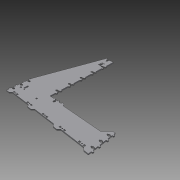
# Autodesk Inventor part: frame_left
Saved by Autodesk Inventor 2014 (Build 180170000, 170)
## iProperties
Created: 2013-12-03
Part Number: frame_left
Material: Generic
Document SubType Name: Modeling
Designer: buben
Density: 1 g/cm^3
Appearance: Default
Author: buben
Autodesk Inventor part; units mm, degrees
ref_plane "YZ Plane" through (0, 0, 0) normal (1, 0, 0) x (0, 1, 0)
ref_plane "XZ Plane" through (0, 0, 0) normal (0, 1, 0) x (-1, 0, 0)
ref_plane "XY Plane" through (0, 0, 0) normal (0, 0, 1) x (1, 0, 0)
sketch "Sketch1" plane through (0, 0, 0) normal (0, 0, 1) x (1, 0, 0)
  line L0 (0, 0) -> (489, 0)
  line L1 (489, 0) -> (489, 120)
  line L2 (0, 0) -> (0, 120)
  line L3 (0, 120) -> (111.5, 494)
  line L4 (111.5, 494) -> (161.5, 494)
  line L5 (161.5, 494) -> (161.5, 94)
  line L6 (489, 120) -> (479, 120)
  line L7 (479, 120) -> (449, 90)
  line L8 (449, 90) -> (251.5, 90)
  line L9 (251.5, 90) -> (241.5, 100)
  line L10 (241.5, 100) -> (231.5, 100)
  line L11 (231.5, 100) -> (231.5, 94)
  line L12 (231.5, 94) -> (161.5, 94)
  point P0 (244.5, 0)
  dimension "d0" = 489
  dimension "d1" = 83
  dimension "d2" = 120
  dimension "d3" = 45
  dimension "d5" = 6
  dimension "d6" = 70
  dimension "d7" = 10
  dimension "d8" = 10
  dimension "d9" = 50
  dimension "d10" = 494
  dimension "d13" = 10
  dimension "d15" = 20
  constraints: 26 end point, 7 perpendicular, 3 parallel, 1 horizontal, 1 horizontal alignment, 1 midpoint
  measures "d0" distance of L0.start L0.end
  measures "d1" distance from line of L5 point (244.5, 0)
  measures "d2" distance of L0.start L2.end
  measures "d3" angle of L6 L7
  measures "d5" distance of L10.end L11.end
  measures "d6" distance of L11.end L5.end
  measures "d7" distance of L1.end L6.end
  measures "d8" distance of L9.end L10.end
  measures "d9" distance of L3.end L4.end
  measures "d10" distance between parallel lines of L0 L4
  measures "d13" distance between parallel lines of L8 L10
  measures "d15" vertical distance of L2.end L10.end
extrude "Extrusion1" add sketch "Sketch1" along normal blind 6
sketch "Sketch2" plane through (0, 0, 6) normal (0, 0, 1) x (1, 0, 0)
  line L0 (0, 0) -> (489, 0) projected
  line L1 (489, 0) -> (489, 120) projected
  line L2 (251.5, 90) -> (241.5, 100) projected
  line L3 (489, 20.75) -> (489, 16.25)
  line L4 (472.7, 16.25) -> (472.7, 20.75)
  line L5 (476.7, 23.25) -> (484, 23.25)
  line L6 (484, 13.75) -> (476.7, 13.75)
  line L7 (472.7, 20.75) -> (476.7, 20.75)
  line L8 (484, 20.75) -> (489, 20.75)
  line L9 (489, 16.25) -> (484, 16.25)
  line L10 (476.7, 16.25) -> (472.7, 16.25)
  line L11 (476.7, 13.75) -> (476.7, 16.25)
  line L12 (476.7, 20.75) -> (476.7, 23.25)
  line L13 (484, 23.25) -> (484, 20.75)
  line L14 (484, 16.25) -> (484, 13.75)
  line L15 (489, 98.75) -> (489, 94.25)
  line L16 (472.7, 94.25) -> (472.7, 98.75)
  line L17 (476.7, 101.25) -> (484, 101.25)
  line L18 (484, 91.75) -> (476.7, 91.75)
  line L19 (472.7, 98.75) -> (476.7, 98.75)
  line L20 (484, 98.75) -> (489, 98.75)
  line L21 (489, 94.25) -> (484, 94.25)
  line L22 (476.7, 94.25) -> (472.7, 94.25)
  line L23 (476.7, 91.75) -> (476.7, 94.25)
  line L24 (476.7, 98.75) -> (476.7, 101.25)
  line L25 (484, 101.25) -> (484, 98.75)
  line L26 (484, 94.25) -> (484, 91.75)
  line L27 (489, 59.75) -> (489, 55.25)
  line L28 (472.7, 55.25) -> (472.7, 59.75)
  line L29 (476.7, 62.25) -> (484, 62.25)
  line L30 (484, 52.75) -> (476.7, 52.75)
  line L31 (472.7, 59.75) -> (476.7, 59.75)
  line L32 (484, 59.75) -> (489, 59.75)
  line L33 (489, 55.25) -> (484, 55.25)
  line L34 (476.7, 55.25) -> (472.7, 55.25)
  line L35 (476.7, 52.75) -> (476.7, 55.25)
  line L36 (476.7, 59.75) -> (476.7, 62.25)
  line L37 (484, 62.25) -> (484, 59.75)
  line L38 (484, 55.25) -> (484, 52.75)
  line L39 (244.5, 0) -> (244.5, 97) construction
  line L40 (0, 20.75) -> (0, 16.25)
  line L41 (16.3, 16.25) -> (16.3, 20.75)
  line L42 (12.3, 23.25) -> (5, 23.25)
  line L43 (5, 13.75) -> (12.3, 13.75)
  line L44 (16.3, 20.75) -> (12.3, 20.75)
  line L45 (5, 20.75) -> (0, 20.75)
  line L46 (0, 16.25) -> (5, 16.25)
  line L47 (12.3, 16.25) -> (16.3, 16.25)
  line L48 (12.3, 13.75) -> (12.3, 16.25)
  line L49 (12.3, 20.75) -> (12.3, 23.25)
  line L50 (5, 23.25) -> (5, 20.75)
  line L51 (5, 16.25) -> (5, 13.75)
  line L52 (16.3, 98.75) -> (12.3, 98.75)
  line L53 (16.3, 94.25) -> (16.3, 98.75)
  line L54 (12.3, 94.25) -> (16.3, 94.25)
  line L55 (12.3, 98.75) -> (12.3, 101.25)
  line L56 (12.3, 91.75) -> (12.3, 94.25)
  line L57 (12.3, 101.25) -> (5, 101.25)
  line L58 (5, 94.25) -> (5, 91.75)
  line L59 (5, 91.75) -> (12.3, 91.75)
  line L60 (5, 98.75) -> (0, 98.75)
  line L61 (0, 98.75) -> (0, 94.25)
  line L62 (0, 94.25) -> (5, 94.25)
  line L63 (5, 101.25) -> (5, 98.75)
  line L64 (12.3, 59.75) -> (12.3, 62.25)
  line L65 (16.3, 59.75) -> (12.3, 59.75)
  line L66 (16.3, 55.25) -> (16.3, 59.75)
  line L67 (12.3, 55.25) -> (16.3, 55.25)
  line L68 (12.3, 52.75) -> (12.3, 55.25)
  line L69 (12.3, 62.25) -> (5, 62.25)
  line L70 (5, 52.75) -> (12.3, 52.75)
  line L71 (5, 55.25) -> (5, 52.75)
  line L72 (5, 62.25) -> (5, 59.75)
  line L73 (0, 55.25) -> (5, 55.25)
  line L74 (5, 59.75) -> (0, 59.75)
  line L75 (0, 59.75) -> (0, 55.25)
  point P0 (472.7, 18.5)
  point P1 (480.35, 23.25)
  point P2 (472.7, 96.5)
  point P3 (480.35, 101.25)
  point P4 (472.7, 57.5)
  point P5 (480.35, 62.25)
  point P6 (16.3, 18.5)
  point P7 (8.65, 23.25)
  point P8 (16.3, 96.5)
  point P9 (8.65, 101.25)
  point P10 (16.3, 57.5)
  point P11 (8.65, 62.25)
  dimension "d16" = 4.5
  dimension "d17" = 2.5
  dimension "d18" = 2.5
  dimension "d19" = 4
  dimension "d20" = 7.3
  dimension "d21" = 5
  dimension "d23" = 4.5
  dimension "d24" = 2.5
  dimension "d25" = 2.5
  dimension "d26" = 4
  dimension "d27" = 7.3
  dimension "d28" = 5
  dimension "d30" = 4.5
  dimension "d31" = 2.5
  dimension "d32" = 2.5
  dimension "d33" = 4
  dimension "d34" = 7.3
  dimension "d35" = 5
  dimension "d40" = 18.5
  dimension "d41" = 39
  dimension "d42" = 39
  constraints: 146 end point, 42 symmetric about line, 30 parallel, 15 collinear, 13 perpendicular, 9 horizontal, 7 midpoint, 1 point on line
  measures "d16" distance of L4.start L4.end
  measures "d17" distance of L7.end L5.start
  measures "d18" distance of L6.end L10.start
  measures "d19" distance of L10.start L4.start
  measures "d20" distance of L6.start L6.end
  measures "d21" distance of L3.end L9.end
  measures "d23" distance of L16.start L19.start
  measures "d24" distance of L19.end L24.end
  measures "d25" distance of L23.start L22.start
  measures "d26" distance of L22.start L16.start
  measures "d27" distance of L26.end L23.start
  measures "d28" distance of L15.end L26.start
  measures "d30" distance of L28.start L31.start
  measures "d31" distance of L36.start L36.end
  measures "d32" distance of L35.start L34.start
  measures "d33" distance of L34.start L28.start
  measures "d34" distance of L30.start L35.start
  measures "d35" distance of L33.start L38.start
  measures "d40" distance from line of L0 point (472.7, 18.5)
  measures "d41" distance of point (472.7, 57.5) point (472.7, 18.5)
  measures "d42" distance of point (472.7, 57.5) point (472.7, 96.5)
extrude "Extrusion2" cut sketch "Sketch2" against normal through all
sketch "Sketch4" plane through (0, 0, 6) normal (0, 0, 1) x (1, 0, 0)
  line L0 (0, 16.25) -> (0, 0) projected
  line L1 (489, 0) -> (489, 16.25) projected
  line L2 (472.7, 16.25) -> (472.7, 20.75) projected
  line L3 (489, 20.75) -> (489, 55.25) projected
  line L4 (472.7, 55.25) -> (472.7, 59.75) projected
  line L5 (489, 59.75) -> (489, 94.25) projected
  line L6 (472.7, 94.25) -> (472.7, 98.75) projected
  line L7 (489, 98.75) -> (489, 120) projected
  line L8 (0, 120) -> (0, 98.75) projected
  line L9 (0, 94.25) -> (0, 59.75) projected
  line L10 (0, 55.25) -> (0, 20.75) projected
  line L11 (0, 112) -> (-4, 112)
  line L12 (-6, 110) -> (-6, 106)
  line L13 (-4, 104) -> (0, 104)
  line L14 (0, 104) -> (0, 112)
  line L15 (0, 81) -> (-4, 81)
  line L16 (-6, 79) -> (-6, 75)
  line L17 (-4, 73) -> (0, 73)
  line L18 (0, 73) -> (0, 81)
  line L19 (0, 42) -> (-4, 42)
  line L20 (-6, 40) -> (-6, 36)
  line L21 (-4, 34) -> (0, 34)
  line L22 (0, 34) -> (0, 42)
  line L23 (0, 11) -> (-4, 11)
  line L24 (-6, 9) -> (-6, 5)
  line L25 (-4, 3) -> (0, 3)
  line L26 (0, 3) -> (0, 11)
  line L27 (489, 112) -> (493, 112)
  line L28 (495, 110) -> (495, 106)
  line L29 (493, 104) -> (489, 104)
  line L30 (489, 104) -> (489, 112)
  line L31 (489, 81) -> (493, 81)
  line L32 (495, 79) -> (495, 75)
  line L33 (493, 73) -> (489, 73)
  line L34 (489, 73) -> (489, 81)
  line L35 (489, 42) -> (493, 42)
  line L36 (495, 40) -> (495, 36)
  line L37 (493, 34) -> (489, 34)
  line L38 (489, 34) -> (489, 42)
  line L39 (489, 11) -> (493, 11)
  line L40 (495, 9) -> (495, 5)
  line L41 (493, 3) -> (489, 3)
  line L42 (489, 3) -> (489, 11)
  arc A0 (-6, 5) -> (-4, 3) centre (-4, 5) ccw
  arc A1 (-4, 11) -> (-6, 9) centre (-4, 9) ccw
  arc A2 (-6, 36) -> (-4, 34) centre (-4, 36) ccw
  arc A3 (-4, 42) -> (-6, 40) centre (-4, 40) ccw
  arc A4 (-6, 75) -> (-4, 73) centre (-4, 75) ccw
  arc A5 (-4, 81) -> (-6, 79) centre (-4, 79) ccw
  arc A6 (-6, 106) -> (-4, 104) centre (-4, 106) ccw
  arc A7 (-4, 112) -> (-6, 110) centre (-4, 110) ccw
  arc A8 (495, 110) -> (493, 112) centre (493, 110) ccw
  arc A9 (493, 104) -> (495, 106) centre (493, 106) ccw
  arc A10 (495, 79) -> (493, 81) centre (493, 79) ccw
  arc A11 (493, 73) -> (495, 75) centre (493, 75) ccw
  arc A12 (495, 40) -> (493, 42) centre (493, 40) ccw
  arc A13 (493, 34) -> (495, 36) centre (493, 36) ccw
  arc A14 (495, 9) -> (493, 11) centre (493, 9) ccw
  arc A15 (493, 3) -> (495, 5) centre (493, 5) ccw
  line L43 (489, 20.75) -> (489, 55.25) projected
  point P0 (472.7, 96.5)
  point P1 (472.7, 57.5)
  point P2 (472.7, 18.5)
  point P3 (495, 77)
  point P4 (489, 77)
  point P5 (495, 38)
  point P6 (489, 38)
  dimension "d81" = 2
  dimension "d82" = 8
  dimension "d83" = 8
  dimension "d84" = 8
  dimension "d85" = 8
  dimension "d86" = 7.5
  dimension "d87" = 7.5
  dimension "d88" = 6
  dimension "d89" = 6
  constraints: 64 end point, 32 point on circle, 32 tangent, 16 centre point, 16 parallel, 15 equal radius, 14 collinear, 8 horizontal, 8 perpendicular, 8 point on line, 7 midpoint, 2 horizontal alignment
  measures "d81" radius of A0
  measures "d82" distance between parallel lines of L29 L27
  measures "d83" distance between parallel lines of L33 L31
  measures "d84" distance between parallel lines of L37 L35
  measures "d85" distance between parallel lines of L41 L39
  measures "d86" distance from line of point (472.7, 96.5) L29
  measures "d87" distance from line of point (472.7, 18.5) L39
  measures "d88" distance between parallel lines of L7 L28
  measures "d89" distance between parallel lines of L8 L12
extrude "Extrusion4" add sketch "Sketch4" against normal blind 6
sketch "Sketch5" plane through (0, 0, 6) normal (0, 0, 1) x (1, 0, 0)
  line L0 (231.5, 100) -> (231.5, 94) projected
  line L1 (231.5, 94) -> (161.5, 94) projected
  line L2 (199.75, 94) -> (204.25, 94)
  line L3 (204.25, 77.7) -> (199.75, 77.7)
  line L4 (206.75, 89) -> (206.75, 81.7)
  line L5 (197.25, 81.7) -> (197.25, 89)
  line L6 (204.25, 94) -> (204.25, 89)
  line L7 (204.25, 81.7) -> (204.25, 77.7)
  line L8 (199.75, 77.7) -> (199.75, 81.7)
  line L9 (199.75, 89) -> (199.75, 94)
  line L10 (197.25, 89) -> (199.75, 89)
  line L11 (204.25, 89) -> (206.75, 89)
  line L12 (206.75, 81.7) -> (204.25, 81.7)
  line L13 (199.75, 81.7) -> (197.25, 81.7)
  point P0 (202, 77.7)
  dimension "d92" = 4.5
  dimension "d93" = 2.5
  dimension "d94" = 2.5
  dimension "d95" = 5
  dimension "d96" = 7.3
  dimension "d97" = 4
  dimension "d98" = 29.5
  constraints: 24 end point, 10 parallel, 5 collinear, 4 perpendicular, 3 horizontal, 1 midpoint
  measures "d92" distance of L3.start L3.end
  measures "d93" distance of L8.end L5.start
  measures "d94" distance of L4.end L7.start
  measures "d95" distance of L2.end L6.end
  measures "d96" distance of L4.start L4.end
  measures "d97" distance of L7.start L3.start
  measures "d98" distance from line of L0 point (202, 77.7)
extrude "Extrusion5" cut sketch "Sketch5" against normal blind 6
sketch "Sketch6" plane through (0, 0, 6) normal (0, 0, 1) x (1, 0, 0)
  line L0 (204.25, 77.7) -> (199.75, 77.7) projected
  line L1 (199.75, 94) -> (161.5, 94) projected
  line L2 (231.5, 94) -> (204.25, 94) projected
  line L3 (186.5, 94) -> (194.5, 94)
  line L4 (194.5, 94) -> (194.5, 98)
  line L5 (192.5, 100) -> (188.5, 100)
  line L6 (186.5, 98) -> (186.5, 94)
  line L7 (209.5, 94) -> (217.5, 94)
  line L8 (217.5, 94) -> (217.5, 98)
  line L9 (215.5, 100) -> (211.5, 100)
  line L10 (209.5, 98) -> (209.5, 94)
  arc A0 (188.5, 100) -> (186.5, 98) centre (188.5, 98) ccw
  arc A1 (194.5, 98) -> (192.5, 100) centre (192.5, 98) ccw
  arc A2 (211.5, 100) -> (209.5, 98) centre (211.5, 98) ccw
  arc A3 (217.5, 98) -> (215.5, 100) centre (215.5, 98) ccw
  point P0 (202, 77.7)
  dimension "d101" = 2
  dimension "d102" = 15
  dimension "d103" = 8
  dimension "d104" = 8
  dimension "d105" = 7.5
  dimension "d106" = 6
  constraints: 16 end point, 8 point on circle, 8 tangent, 4 centre point, 4 parallel, 3 equal radius, 2 horizontal, 2 perpendicular, 2 point on line, 1 collinear, 1 midpoint
  measures "d101" radius of A0
  measures "d102" distance between parallel lines of L4 L10
  measures "d103" distance between parallel lines of L6 L4
  measures "d104" distance between parallel lines of L8 L10
  measures "d105" distance from line of point (202, 77.7) L4
  measures "d106" distance between parallel lines of L1 L5
extrude "Extrusion6" add sketch "Sketch6" against normal blind 6
sketch "Sketch7" plane through (0, 0, 6) normal (0, 0, 1) x (1, 0, 0)
  line L0 (161.5, 94) -> (161.5, 494) projected
  line L1 (161.5, 494) -> (111.5, 494) projected
  line L2 (134, 446) -> (126, 446)
  line L3 (126, 446) -> (126, 440)
  line L4 (126, 440) -> (134, 440)
  line L5 (134, 440) -> (134, 446)
  circle A0 centre (141.5, 443) radius 2.25
  point P0 (134, 443)
  dimension "d109" = 6
  dimension "d110" = 8
  dimension "d118" = 7.5
  dimension "d119" = 20
  dimension "d120" = 48
  dimension "d121" = 4.5
  constraints: 8 end point, 2 parallel, 1 centre point, 1 horizontal, 1 horizontal alignment, 1 midpoint, 1 perpendicular
  measures "d109" distance of L2.end L3.end
  measures "d110" distance of L2.start L2.end
  measures "d118" distance from line of A0.centre L5
  measures "d119" distance from line of L0 A0.centre
  measures "d120" distance between parallel lines of L1 L2
  measures "d121" diameter of A0
extrude "Extrusion8" cut sketch "Sketch7" against normal blind 6
sketch "Sketch8" plane through (0, 0, 6) normal (0, 0, 1) x (1, 0, 0)
  line L0 (161.5, 494) -> (117.5, 494)
  line L1 (117.5, 494) -> (117.5, 488)
  line L2 (117.5, 488) -> (161.5, 488)
  line L3 (161.5, 488) -> (161.5, 494)
  point P0 (111.5, 494)
  dimension "d124" = 6
  dimension "d125" = 6
  constraints: 8 end point, 2 parallel, 1 horizontal, 1 perpendicular
  measures "d124" distance from line of point (111.5, 494) L1
  measures "d125" distance of L0.end L1.end
extrude "Extrusion9" cut sketch "Sketch8" against normal through all
sketch "Sketch9" plane through (0, 0, 6) normal (0, 0, 1) x (1, 0, 0)
  line L0 (161.5, 94) -> (161.5, 488) projected
  line L1 (161.5, 420.75) -> (161.5, 416.25)
  line L2 (145.2, 416.25) -> (145.2, 420.75)
  line L3 (149.2, 423.25) -> (156.5, 423.25)
  line L4 (156.5, 413.75) -> (149.2, 413.75)
  line L5 (156.5, 423.25) -> (156.5, 420.75)
  line L6 (156.5, 416.25) -> (156.5, 413.75)
  line L7 (149.2, 413.75) -> (149.2, 416.25)
  line L8 (149.2, 420.75) -> (149.2, 423.25)
  line L9 (145.2, 420.75) -> (149.2, 420.75)
  line L10 (156.5, 420.75) -> (161.5, 420.75)
  line L11 (161.5, 416.25) -> (156.5, 416.25)
  line L12 (149.2, 416.25) -> (145.2, 416.25)
  line L13 (161.5, 350.75) -> (161.5, 346.25)
  line L14 (145.2, 346.25) -> (145.2, 350.75)
  line L15 (149.2, 353.25) -> (156.5, 353.25)
  line L16 (156.5, 343.75) -> (149.2, 343.75)
  line L17 (156.5, 353.25) -> (156.5, 350.75)
  line L18 (156.5, 346.25) -> (156.5, 343.75)
  line L19 (149.2, 343.75) -> (149.2, 346.25)
  line L20 (149.2, 350.75) -> (149.2, 353.25)
  line L21 (145.2, 350.75) -> (149.2, 350.75)
  line L22 (156.5, 350.75) -> (161.5, 350.75)
  line L23 (161.5, 346.25) -> (156.5, 346.25)
  line L24 (149.2, 346.25) -> (145.2, 346.25)
  line L25 (161.5, 280.75) -> (161.5, 276.25)
  line L26 (145.2, 276.25) -> (145.2, 280.75)
  line L27 (149.2, 283.25) -> (156.5, 283.25)
  line L28 (156.5, 273.75) -> (149.2, 273.75)
  line L29 (156.5, 283.25) -> (156.5, 280.75)
  line L30 (156.5, 276.25) -> (156.5, 273.75)
  line L31 (149.2, 273.75) -> (149.2, 276.25)
  line L32 (149.2, 280.75) -> (149.2, 283.25)
  line L33 (145.2, 280.75) -> (149.2, 280.75)
  line L34 (156.5, 280.75) -> (161.5, 280.75)
  line L35 (161.5, 276.25) -> (156.5, 276.25)
  line L36 (149.2, 276.25) -> (145.2, 276.25)
  line L37 (161.5, 210.75) -> (161.5, 206.25)
  line L38 (145.2, 206.25) -> (145.2, 210.75)
  line L39 (149.2, 213.25) -> (156.5, 213.25)
  line L40 (156.5, 203.75) -> (149.2, 203.75)
  line L41 (156.5, 213.25) -> (156.5, 210.75)
  line L42 (156.5, 206.25) -> (156.5, 203.75)
  line L43 (149.2, 203.75) -> (149.2, 206.25)
  line L44 (149.2, 210.75) -> (149.2, 213.25)
  line L45 (145.2, 210.75) -> (149.2, 210.75)
  line L46 (156.5, 210.75) -> (161.5, 210.75)
  line L47 (161.5, 206.25) -> (156.5, 206.25)
  line L48 (149.2, 206.25) -> (145.2, 206.25)
  line L49 (161.5, 140.75) -> (161.5, 136.25)
  line L50 (145.2, 136.25) -> (145.2, 140.75)
  line L51 (149.2, 143.25) -> (156.5, 143.25)
  line L52 (156.5, 133.75) -> (149.2, 133.75)
  line L53 (156.5, 143.25) -> (156.5, 140.75)
  line L54 (156.5, 136.25) -> (156.5, 133.75)
  line L55 (149.2, 133.75) -> (149.2, 136.25)
  line L56 (149.2, 140.75) -> (149.2, 143.25)
  line L57 (145.2, 140.75) -> (149.2, 140.75)
  line L58 (156.5, 140.75) -> (161.5, 140.75)
  line L59 (161.5, 136.25) -> (156.5, 136.25)
  line L60 (149.2, 136.25) -> (145.2, 136.25)
  point P0 (117.5, 494)
  point P1 (145.2, 418.5)
  point P2 (145.2, 348.5)
  point P3 (145.2, 278.5)
  point P4 (145.2, 208.5)
  point P5 (145.2, 138.5)
  dimension "d128" = 4.5
  dimension "d129" = 2.5
  dimension "d130" = 2.5
  dimension "d131" = 5
  dimension "d132" = 7.3
  dimension "d133" = 4
  dimension "d134" = 75.5
  dimension "d137" = 70
  constraints: 120 end point, 10 parallel, 5 collinear, 4 perpendicular, 3 horizontal, 1 midpoint, 1 vertical, 100 other
  measures "d128" distance of L2.start L2.end
  measures "d129" distance of L8.start L3.start
  measures "d130" distance of L4.end L7.end
  measures "d131" distance of L1.end L6.start
  measures "d132" distance of L4.start L4.end
  measures "d133" distance of L7.end L2.start
  measures "d134" vertical distance of point (117.5, 494) point (145.2, 418.5)
  measures "d137" distance of L1.end L23.start
extrude "Extrusion10" cut sketch "Sketch9" against normal through all
sketch "Sketch10" plane through (0, 0, 6) normal (0, 0, 1) x (1, 0, 0)
  line L0 (161.5, 350.75) -> (161.5, 416.25) projected
  line L1 (145.2, 416.25) -> (145.2, 420.75) projected
  line L2 (161.5, 420.75) -> (161.5, 488) projected
  line L3 (161.5, 434) -> (165.5, 434)
  line L4 (167.5, 432) -> (167.5, 428)
  line L5 (165.5, 426) -> (161.5, 426)
  line L6 (161.5, 426) -> (161.5, 434)
  line L7 (161.5, 411) -> (165.5, 411)
  line L8 (167.5, 409) -> (167.5, 405)
  line L9 (165.5, 403) -> (161.5, 403)
  line L10 (161.5, 403) -> (161.5, 411)
  arc A0 (167.5, 432) -> (165.5, 434) centre (165.5, 432) ccw
  arc A1 (165.5, 426) -> (167.5, 428) centre (165.5, 428) ccw
  arc A2 (167.5, 409) -> (165.5, 411) centre (165.5, 409) ccw
  arc A3 (165.5, 403) -> (167.5, 405) centre (165.5, 405) ccw
  line L11 (161.5, 364) -> (165.5, 364)
  line L12 (167.5, 362) -> (167.5, 358)
  line L13 (165.5, 356) -> (161.5, 356)
  line L14 (161.5, 356) -> (161.5, 364)
  line L15 (161.5, 341) -> (165.5, 341)
  line L16 (167.5, 339) -> (167.5, 335)
  line L17 (165.5, 333) -> (161.5, 333)
  line L18 (161.5, 333) -> (161.5, 341)
  arc A4 (167.5, 362) -> (165.5, 364) centre (165.5, 362) ccw
  arc A5 (165.5, 356) -> (167.5, 358) centre (165.5, 358) ccw
  arc A6 (167.5, 339) -> (165.5, 341) centre (165.5, 339) ccw
  arc A7 (165.5, 333) -> (167.5, 335) centre (165.5, 335) ccw
  line L19 (161.5, 294) -> (165.5, 294)
  line L20 (167.5, 292) -> (167.5, 288)
  line L21 (165.5, 286) -> (161.5, 286)
  line L22 (161.5, 286) -> (161.5, 294)
  line L23 (161.5, 271) -> (165.5, 271)
  line L24 (167.5, 269) -> (167.5, 265)
  line L25 (165.5, 263) -> (161.5, 263)
  line L26 (161.5, 263) -> (161.5, 271)
  arc A8 (167.5, 292) -> (165.5, 294) centre (165.5, 292) ccw
  arc A9 (165.5, 286) -> (167.5, 288) centre (165.5, 288) ccw
  arc A10 (167.5, 269) -> (165.5, 271) centre (165.5, 269) ccw
  arc A11 (165.5, 263) -> (167.5, 265) centre (165.5, 265) ccw
  line L27 (161.5, 224) -> (165.5, 224)
  line L28 (167.5, 222) -> (167.5, 218)
  line L29 (165.5, 216) -> (161.5, 216)
  line L30 (161.5, 216) -> (161.5, 224)
  line L31 (161.5, 201) -> (165.5, 201)
  line L32 (167.5, 199) -> (167.5, 195)
  line L33 (165.5, 193) -> (161.5, 193)
  line L34 (161.5, 193) -> (161.5, 201)
  arc A12 (167.5, 222) -> (165.5, 224) centre (165.5, 222) ccw
  arc A13 (165.5, 216) -> (167.5, 218) centre (165.5, 218) ccw
  arc A14 (167.5, 199) -> (165.5, 201) centre (165.5, 199) ccw
  arc A15 (165.5, 193) -> (167.5, 195) centre (165.5, 195) ccw
  line L35 (161.5, 154) -> (165.5, 154)
  line L36 (167.5, 152) -> (167.5, 148)
  line L37 (165.5, 146) -> (161.5, 146)
  line L38 (161.5, 146) -> (161.5, 154)
  line L39 (161.5, 131) -> (165.5, 131)
  line L40 (167.5, 129) -> (167.5, 125)
  line L41 (165.5, 123) -> (161.5, 123)
  line L42 (161.5, 123) -> (161.5, 131)
  arc A16 (167.5, 152) -> (165.5, 154) centre (165.5, 152) ccw
  arc A17 (165.5, 146) -> (167.5, 148) centre (165.5, 148) ccw
  arc A18 (167.5, 129) -> (165.5, 131) centre (165.5, 129) ccw
  arc A19 (165.5, 123) -> (167.5, 125) centre (165.5, 125) ccw
  point P0 (145.2, 418.5)
  dimension "d144" = 2
  dimension "d145" = 8
  dimension "d146" = 8
  dimension "d147" = 6
  dimension "d148" = 15
  dimension "d149" = 7.5
  dimension "d152" = 70
  constraints: 80 end point, 40 point on circle, 20 centre point, 8 tangent, 4 parallel, 3 equal radius, 2 horizontal, 2 perpendicular, 2 point on line, 1 collinear, 1 midpoint, 1 vertical, 112 other
  measures "d144" radius of A0
  measures "d145" distance between parallel lines of L9 L7
  measures "d146" distance between parallel lines of L5 L3
  measures "d147" distance between parallel lines of L6 L4
  measures "d148" distance between parallel lines of L5 L7
  measures "d149" distance from line of L5 point (145.2, 418.5)
  measures "d152" distance of A1.centre A5.centre
extrude "Extrusion11" add sketch "Sketch10" against normal blind 6
sketch "Sketch11" plane through (0, 0, 6) normal (0, 0, 1) x (1, 0, 0)
  line L0 (161.5, 488) -> (117.5, 488) projected
  line L1 (117.5, 488) -> (117.5, 494) projected
  line L2 (127.25, 488) -> (131.75, 488)
  line L3 (131.75, 471.7) -> (127.25, 471.7)
  line L4 (134.25, 483) -> (134.25, 475.7)
  line L5 (124.75, 475.7) -> (124.75, 483)
  line L6 (124.75, 483) -> (127.25, 483)
  line L7 (131.75, 483) -> (134.25, 483)
  line L8 (134.25, 475.7) -> (131.75, 475.7)
  line L9 (127.25, 475.7) -> (124.75, 475.7)
  line L10 (127.25, 471.7) -> (127.25, 475.7)
  line L11 (127.25, 483) -> (127.25, 488)
  line L12 (131.75, 488) -> (131.75, 483)
  line L13 (131.75, 475.7) -> (131.75, 471.7)
  point P0 (129.5, 471.7)
  dimension "d159" = 4.5
  dimension "d160" = 2.5
  dimension "d161" = 2.5
  dimension "d162" = 5
  dimension "d163" = 7.3
  dimension "d164" = 4
  dimension "d165" = 12
  constraints: 24 end point, 10 parallel, 5 collinear, 4 perpendicular, 3 horizontal, 1 midpoint
  measures "d159" distance of L3.start L3.end
  measures "d160" distance of L4.end L8.end
  measures "d161" distance of L9.start L5.start
  measures "d162" distance of L2.end L7.start
  measures "d163" distance of L4.start L4.end
  measures "d164" distance of L8.end L3.start
  measures "d165" distance from line of L1 point (129.5, 471.7)
extrude "Extrusion12" cut sketch "Sketch11" against normal blind 6
sketch "Sketch12" plane through (0, 0, 6) normal (0, 0, 1) x (1, 0, 0)
  line L0 (0, 0) -> (489, 0) projected
  line L1 (30, 9) -> (38, 9)
  line L2 (38, 9) -> (38, 3)
  line L3 (38, 3) -> (30, 3)
  line L4 (30, 3) -> (30, 9)
  line L5 (53, 9) -> (61, 9)
  line L6 (61, 9) -> (61, 3)
  line L7 (61, 3) -> (53, 3)
  line L8 (53, 3) -> (53, 9)
  line L9 (38, 9) -> (53, 3) construction
  line L10 (53, 9) -> (38, 3) construction
  circle A0 centre (45.5, 6) radius 2.25
  line L11 (129.5, 9) -> (137.5, 9)
  line L12 (137.5, 9) -> (137.5, 3)
  line L13 (137.5, 3) -> (129.5, 3)
  line L14 (129.5, 3) -> (129.5, 9)
  line L15 (152.5, 9) -> (160.5, 9)
  line L16 (160.5, 9) -> (160.5, 3)
  line L17 (160.5, 3) -> (152.5, 3)
  line L18 (152.5, 3) -> (152.5, 9)
  line L19 (137.5, 9) -> (152.5, 3) construction
  line L20 (152.5, 9) -> (137.5, 3) construction
  circle A1 centre (145, 6) radius 2.25
  line L21 (328.5, 9) -> (336.5, 9)
  line L22 (336.5, 9) -> (336.5, 3)
  line L23 (336.5, 3) -> (328.5, 3)
  line L24 (328.5, 3) -> (328.5, 9)
  line L25 (351.5, 9) -> (359.5, 9)
  line L26 (359.5, 9) -> (359.5, 3)
  line L27 (359.5, 3) -> (351.5, 3)
  line L28 (351.5, 3) -> (351.5, 9)
  line L29 (336.5, 9) -> (351.5, 3) construction
  line L30 (351.5, 9) -> (336.5, 3) construction
  circle A2 centre (344, 6) radius 2.25
  line L31 (428, 9) -> (436, 9)
  line L32 (436, 9) -> (436, 3)
  line L33 (436, 3) -> (428, 3)
  line L34 (428, 3) -> (428, 9)
  line L35 (451, 9) -> (459, 9)
  line L36 (459, 9) -> (459, 3)
  line L37 (459, 3) -> (451, 3)
  line L38 (451, 3) -> (451, 9)
  line L39 (436, 9) -> (451, 3) construction
  line L40 (451, 9) -> (436, 3) construction
  circle A3 centre (443.5, 6) radius 2.25
  line L41 (229, 9) -> (237, 9)
  line L42 (237, 9) -> (237, 3)
  line L43 (237, 3) -> (229, 3)
  line L44 (229, 3) -> (229, 9)
  line L45 (252, 9) -> (260, 9)
  line L46 (260, 9) -> (260, 3)
  line L47 (260, 3) -> (252, 3)
  line L48 (252, 3) -> (252, 9)
  line L49 (237, 9) -> (252, 3) construction
  line L50 (252, 9) -> (237, 3) construction
  circle A4 centre (244.5, 6) radius 2.25
  line L51 (61, 6) -> (129.5, 6) construction
  line L52 (160.5, 6) -> (229, 6) construction
  line L53 (260, 6) -> (328.5, 6) construction
  line L54 (359.5, 6) -> (428, 6) construction
  point P0 (145, 6)
  point P1 (344, 6)
  dimension "d168" = 8
  dimension "d169" = 8
  dimension "d170" = 6
  dimension "d171" = 15
  dimension "d172" = 4.5
  dimension "d173" = 8
  dimension "d174" = 8
  dimension "d175" = 6
  dimension "d176" = 15
  dimension "d177" = 4.5
  dimension "d178" = 8
  dimension "d179" = 8
  dimension "d180" = 6
  dimension "d181" = 15
  dimension "d182" = 4.5
  dimension "d183" = 8
  dimension "d184" = 8
  dimension "d185" = 6
  dimension "d186" = 15
  dimension "d187" = 4.5
  dimension "d188" = 8
  dimension "d189" = 8
  dimension "d190" = 6
  dimension "d191" = 15
  dimension "d192" = 4.5
  dimension "d198" = 3
  dimension "d206" = 30
  dimension "d207" = 30
  constraints: 108 end point, 20 parallel, 15 midpoint, 13 collinear, 10 horizontal, 10 perpendicular, 5 centre point, 4 horizontal alignment
  measures "d168" distance of L1.start L1.end
  measures "d169" distance of L5.start L5.end
  measures "d170" distance of L3.end L1.start
  measures "d171" distance between parallel lines of L8 L2
  measures "d172" diameter of A0
  measures "d173" distance of L11.start L11.end
  measures "d174" distance of L15.start L15.end
  measures "d175" distance of L14.start L11.start
  measures "d176" distance between parallel lines of L18 L12
  measures "d177" diameter of A1
  measures "d178" distance of L21.start L21.end
  measures "d179" distance of L25.start L25.end
  measures "d180" distance of L24.start L21.start
  measures "d181" distance between parallel lines of L28 L22
  measures "d182" diameter of A2
  measures "d183" distance of L31.start L31.end
  measures "d184" distance of L35.start L35.end
  measures "d185" distance of L34.start L31.start
  measures "d186" distance between parallel lines of L38 L32
  measures "d187" diameter of A3
  measures "d188" distance of L41.start L41.end
  measures "d189" distance of L45.start L45.end
  measures "d190" distance of L44.start L41.start
  measures "d191" distance between parallel lines of L48 L42
  measures "d192" diameter of A4
  measures "d198" distance between parallel lines of L0 L3
  measures "d206" distance from line of L0.end L36
  measures "d207" distance from line of L0.start L4
extrude "Extrusion13" cut sketch "Sketch12" against normal through all
sketch "Sketch13" plane through (0, 0, 6) normal (0, 0, 1) x (1, 0, 0)
  line L0 (0, 0) -> (489, 0) projected
  line L1 (134, 440) -> (126, 440) projected
  line L2 (0, 0) -> (0, -10)
  line L3 (0, -10) -> (20, -10)
  line L4 (20, -10) -> (30, 0)
  line L5 (146.3333, 0) -> (156.3333, -10)
  line L6 (156.3333, -10) -> (176.3333, -10)
  line L7 (176.3333, -10) -> (186.3333, 0)
  line L8 (302.6667, 0) -> (312.6667, -10)
  line L9 (312.6667, -10) -> (332.6667, -10)
  line L10 (332.6667, -10) -> (342.6667, 0)
  line L11 (489, 0) -> (489, -10)
  line L12 (489, -10) -> (469, -10)
  line L13 (469, -10) -> (459, 0)
  line L14 (20, -10) -> (156.3333, -10) construction
  line L15 (176.3333, -10) -> (312.6667, -10) construction
  line L16 (332.6667, -10) -> (469, -10) construction
  dimension "d201" = 10
  dimension "d202" = 20
  dimension "d203" = 45
  constraints: 30 end point, 13 collinear, 9 perpendicular, 6 point on line
  measures "d201" distance of L0.start L2.end
  measures "d202" distance of L2.end L3.end
  measures "d203" angle of L3 L4
extrude "Extrusion14" add sketch "Sketch13" against normal blind 6
sketch "Sketch14" plane through (0, 0, 6) normal (0, 0, 1) x (1, 0, 0)
  line L0 (252, 3) -> (252, 9) projected
  line L1 (0, 73) -> (0, 59.75) projected
  line L2 (30, 0) -> (146.3333, 0) projected
  line L3 (40, 69) -> (40, 54) construction
  line L4 (36, 69) -> (36, 54)
  line L5 (44, 54) -> (44, 69)
  arc A0 (44, 69) -> (36, 69) centre (40, 69) ccw
  arc A1 (36, 54) -> (44, 54) centre (40, 54) ccw
  point P0 (0, 0)
  point P1 (40, 61.5)
  dimension "d208" = 15
  dimension "d209" = 8
  dimension "d210" = 54
  dimension "d211" = 40
  constraints: 8 end point, 4 point on circle, 4 tangent, 2 centre point, 2 parallel, 1 midpoint
  measures "d208" distance of L3.start L3.end
  measures "d209" distance between parallel lines of L5 L4
  measures "d210" distance from line of L3.end L2
  measures "d211" distance between parallel lines of L1 L3
extrude "Extrusion15" cut sketch "Sketch14" against normal blind 6
sketch "Sketch15" plane through (0, 0, 6) normal (0, 0, 1) x (1, 0, 0)
  arc A0 (36, 54) -> (44, 54) centre (40, 54) ccw projected
  line L0 (0, 55.25) -> (0, 42) projected
  line L1 (0, 34) -> (0, 20.75) projected
  line L2 (20, 48) -> (28, 48)
  line L3 (28, 48) -> (28, 42)
  line L4 (28, 42) -> (20, 42)
  line L5 (20, 42) -> (20, 48)
  line L6 (133.5, 48) -> (141.5, 48)
  line L7 (141.5, 48) -> (141.5, 42)
  line L8 (141.5, 42) -> (133.5, 42)
  line L9 (133.5, 42) -> (133.5, 48)
  circle A1 centre (50, 45) radius 2.25
  point P0 (0, 0)
  point P1 (28, 45)
  dimension "d214" = 8
  dimension "d215" = 8
  dimension "d216" = 6
  dimension "d217" = 20
  dimension "d218" = 105.5
  dimension "d219" = 6
  dimension "d220" = 4.5
  dimension "d221" = 50
  constraints: 16 end point, 4 parallel, 2 collinear, 2 horizontal, 2 perpendicular, 1 centre point, 1 horizontal alignment, 1 midpoint
  measures "d214" distance of L2.start L2.end
  measures "d215" distance of L6.start L6.end
  measures "d216" distance of L4.end L2.start
  measures "d217" distance between parallel lines of L1 L5
  measures "d218" distance between parallel lines of L9 L3
  measures "d219" distance from line of A0.centre L2
  measures "d220" diameter of A1
  measures "d221" distance from line of L0 A1.centre
extrude "Extrusion16" cut sketch "Sketch15" against normal blind 6
sketch "Sketch16" plane through (0, 0, 6) normal (0, 0, 1) x (1, 0, 0)
  line L0 (251.5, 90) -> (241.5, 100) projected
  line L1 (161.5, 434) -> (161.5, 488) projected
  line L2 (134, 440) -> (126, 440) projected
  line L3 (126.5, 435) -> (138.5, 435) construction
  line L4 (138.5, 435) -> (138.5, 419) construction
  line L5 (138.5, 419) -> (126.5, 419) construction
  line L6 (126.5, 419) -> (126.5, 435) construction
  circle A0 centre (126.5, 419) radius 1.6
  circle A1 centre (138.5, 419) radius 1.6
  circle A2 centre (138.5, 435) radius 1.6
  circle A3 centre (126.5, 435) radius 1.6
  line L7 (130.5, 434) -> (134.5, 434)
  line L8 (139.5, 429) -> (139.5, 425)
  line L9 (134.5, 420) -> (130.5, 420)
  line L10 (125.5, 425) -> (125.5, 429)
  line L11 (125.5, 425) -> (130.5, 420)
  line L12 (134.5, 420) -> (139.5, 425)
  line L13 (139.5, 429) -> (134.5, 434)
  line L14 (130.5, 434) -> (125.5, 429)
  point P0 (0, 0)
  point P1 (132.5, 434)
  point P2 (132.5, 435)
  dimension "d224" = 16
  dimension "d225" = 12
  dimension "d226" = 3.2
  dimension "d227" = 1
  dimension "d228" = 1
  dimension "d229" = 6
  dimension "d230" = 22
  dimension "d231" = 5
  constraints: 24 end point, 9 perpendicular, 5 parallel, 4 centre point, 4 coincident, 3 equal radius, 2 horizontal, 2 midpoint, 1 vertical alignment
  measures "d224" distance of L5.end L3.start
  measures "d225" distance of L3.start L3.end
  measures "d226" diameter of A0
  measures "d227" distance between parallel lines of L3 L7
  measures "d228" distance between parallel lines of L5 L9
  measures "d229" distance between parallel lines of L2 L7
  measures "d230" distance between parallel lines of L1 L8
  measures "d231" horizontal distance of L10.start L9.end
extrude "Extrusion17" cut sketch "Sketch16" against normal blind 6
body "Solid1"
